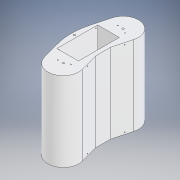
# Autodesk Inventor part: TA001
Saved by Autodesk Inventor 2017 SP1 (Build 210196100, 196)
## iProperties
Created: 2017-09-22
Part Number: TA001
Material: ABS Plastic
Document SubType Name: Modeling
Designer: Zach
Density: 1.06 g/cm^3
Appearance: CR White
Author: Zach
Autodesk Inventor part; units mm, degrees
ref_plane "YZ Plane" through (0, 0, 0) normal (1, 0, 0) x (0, 1, 0)
ref_plane "XZ Plane" through (0, 0, 0) normal (0, 1, 0) x (-1, 0, 0)
ref_plane "XY Plane" through (0, 0, 0) normal (0, 0, 1) x (1, 0, 0)
sketch "Sketch2" plane through (0, 0, 0) normal (0, 1, 0) x (-1, 0, 0)
  circle A0 centre (0, 0) radius 80 construction
  line L0 (77.2741, 20.7055) -> (103.156, -75.8871)
  line L1 (-77.2741, -20.7055) -> (-51.3922, -117.2981)
  line L2 (103.156, -75.8871) -> (-51.3922, -117.2981) construction
  line L3 (103.156, -75.8871) -> (103.156, -235.8871) construction
  line L4 (103.156, -235.8871) -> (-51.3922, -194.476) construction
  line L5 (-51.3922, -117.2981) -> (-51.3922, -194.476)
  circle A1 centre (0, -311.7741) radius 80 construction
  line L6 (-51.3922, -194.476) -> (-77.2741, -291.0686)
  line L7 (103.156, -235.8871) -> (77.2741, -332.4796)
  arc A2 (77.2741, 20.7055) -> (-77.2741, -20.7055) centre (0, 0) ccw
  arc A3 (-77.2741, -291.0686) -> (77.2741, -332.4796) centre (0, -311.7741) ccw
  circle A4 centre (0, 0) radius 5.25
  circle A5 centre (0, -311.7741) radius 5.25
  line L8 (83.156, -49.3871) -> (-29.844, -49.3871)
  line L9 (-29.844, -49.3871) -> (-29.844, -262.3871)
  line L10 (-29.844, -262.3871) -> (83.156, -262.3871)
  line L11 (83.156, -262.3871) -> (83.156, -49.3871)
  arc A6 (103.156, -235.8871) -> (103.156, -75.8871) centre (-201.516, -155.8871) ccw
  circle A7 centre (98.32, -155.8871) radius 5.25
  point P0 (103.156, -155.8871)
  point P1 (83.156, -155.8871)
  dimension "d0" = 160
  dimension "d1" = 100
  dimension "d2" = 100
  dimension "d3" = 160
  dimension "d4" = 160
  dimension "d5" = 160
  dimension "d6" = 75
  dimension "d7" = 75
  dimension "d8" = 160
  dimension "d9" = 100
  dimension "d10" = 100
  dimension "d11" = 10.5
  dimension "d12" = 10.5
  dimension "d13" = 113
  dimension "d14" = 213
  dimension "d15" = 20
  dimension "d39" = 315
  dimension "d40" = 10.5
  dimension "d41" = 15.164
  constraints: 24 end point, 10 point on circle, 8 centre point, 8 tangent, 4 coincident, 2 horizontal alignment, 2 midpoint, 2 parallel, 1 horizontal, 1 perpendicular, 1 vertical
  measures "d0" diameter of A0
  measures "d1" distance of L0.end L0.start
  measures "d2" distance of L1.end L1.start
  measures "d3" distance of L0.end L1.end
  measures "d4" distance of L0.end L3.end
  measures "d5" distance of L3.end L4.end
  measures "d6" angle of L3 L2
  measures "d7" angle of L3 L4
  measures "d8" diameter of A1
  measures "d9" distance of L4.end L6.end
  measures "d10" distance of L3.end L7.end
  measures "d11" diameter of A4
  measures "d12" diameter of A5
  measures "d13" distance of L10.end L9.end
  measures "d14" distance of L9.end L8.end
  measures "d15" distance between parallel lines of L3 L11
  measures "d39" radius of A6
  measures "d40" diameter of A7
  measures "d41" distance from line of L11 A7.centre
extrude "Extrusion1" add sketch "Sketch2" along normal blind 415 contours L0 A6 L7 A3 L6 L5 L1 A2 | A7
sketch "Sketch4" plane through (0, 0, 0) normal (1, 0, 0) x (0, 1, 0)
  line L0 (241.1371, 0) -> (230.6371, 0) construction
  line L1 (215.1815, 0) -> (315.8871, 0) construction
  line L2 (415, -306.5241) -> (415, -317.0241) projected
  line L3 (0, -317.0241) -> (0, -306.5241) projected
  line L4 (415, 5.25) -> (415, -5.25) projected
  line L5 (0, -5.25) -> (0, 5.25) projected
  line L6 (0, -306.5241) -> (415, -306.5241) construction
  line L7 (0, -317.0241) -> (415, -317.0241) construction
  line L8 (0, -5.25) -> (415, -5.25) construction
  line L9 (0, 5.25) -> (415, 5.25) construction
  line L10 (10, -322.5241) -> (40, -322.5241)
  line L11 (40, -322.5241) -> (40, -301.0241)
  line L12 (40, -301.0241) -> (10, -301.0241)
  line L13 (10, -301.0241) -> (10, -322.5241)
  line L14 (40, -10.75) -> (10, -10.75)
  line L15 (10, -10.75) -> (10, 10.75)
  line L16 (10, 10.75) -> (40, 10.75)
  line L17 (40, 10.75) -> (40, -10.75)
  line L18 (80, -322.5241) -> (110, -322.5241)
  line L19 (110, -322.5241) -> (110, -301.0241)
  line L20 (110, -301.0241) -> (80, -301.0241)
  line L21 (80, -301.0241) -> (80, -322.5241)
  line L22 (80, -10.75) -> (110, -10.75)
  line L23 (110, -10.75) -> (110, 10.75)
  line L24 (110, 10.75) -> (80, 10.75)
  line L25 (80, 10.75) -> (80, -10.75)
  point P0 (10, -311.7741)
  point P1 (0, -311.7741)
  point P2 (10, 0)
  point P3 (0, 0)
  dimension "d42" = 30
  dimension "d43" = 21.5
  dimension "d44" = 30
  dimension "d45" = 21.5
  dimension "d46" = 10
  dimension "d47" = 30
  dimension "d48" = 21.5
  dimension "d49" = 40
  dimension "d50" = 30
  dimension "d51" = 21.5
  constraints: 36 end point, 8 parallel, 4 horizontal, 4 horizontal alignment, 4 midpoint, 4 perpendicular, 1 point on line, 1 vertical alignment
  measures "d42" distance of L12.end L11.end
  measures "d43" distance of L11.end L10.end
  measures "d44" distance of L15.end L16.end
  measures "d45" distance of L14.end L15.end
  measures "d46" distance of point (0, -311.774) point (10, -311.774)
  measures "d47" distance of L20.end L19.end
  measures "d48" distance of L19.end L18.end
  measures "d49" distance between parallel lines of L11 L21
  measures "d50" distance of L24.end L23.end
  measures "d51" distance of L23.end L22.end
extrude "Extrusion3" cut sketch "Sketch4" against normal blind 113.156 and the other way blind 20
sketch "Sketch5" plane through (29.844, 0, -49.3871) normal (-1, 0, 0) x (0, 0, 1)
  line L0 (0, 0) -> (-213, 0) construction
  line L1 (0, 0) -> (0, 415) construction
  line L2 (-213, 415) -> (0, 415) construction
  line L3 (-213, 0) -> (-213, 415) construction
  line L4 (-67.911, 0) -> (28.6815, 0) construction
  line L5 (0, 415) -> (-19, 415) construction
  line L6 (-19, 415) -> (-19, 0) construction
  line L7 (-19, 0) -> (0, 0) construction
  line L8 (0, 0) -> (0, 415) construction
  line L9 (-145.089, 415) -> (-241.6815, 415) construction
  line L10 (-213, 0) -> (-194, 0) construction
  line L11 (-194, 0) -> (-194, 415) construction
  line L12 (-194, 415) -> (-213, 415) construction
  line L13 (-213, 415) -> (-213, 0) construction
  circle A0 centre (-203.5, 405) radius 2.5
  circle A1 centre (-203.5, 10) radius 2.5
  circle A2 centre (-9.5, 405) radius 2.5
  circle A3 centre (-9.5, 10) radius 2.5
  point P0 (49.3871, 0)
  point P1 (-203.5, 0)
  point P2 (-203.5, 415)
  point P3 (-9.5, 0)
  point P4 (-9.5, 415)
  dimension "d52" = 19
  dimension "d53" = 19
  dimension "d54" = 5
  dimension "d55" = 10
  dimension "d56" = 5
  dimension "d57" = 10
  dimension "d58" = 5
  dimension "d59" = 5
  dimension "d60" = 10
  dimension "d61" = 10
  constraints: 16 end point, 4 centre point, 4 midpoint, 4 parallel, 4 vertical alignment, 2 horizontal, 2 perpendicular, 2 point on line
  measures "d52" distance of L7.end L6.end
  measures "d53" distance of L12.end L11.end
  measures "d54" diameter of A0
  measures "d55" distance from line of L2 A0.centre
  measures "d56" diameter of A1
  measures "d57" distance from line of L10 A1.centre
  measures "d58" diameter of A2
  measures "d59" diameter of A3
  measures "d60" distance from line of L5 A2.centre
  measures "d61" distance from line of L0 A3.centre
extrude "Extrusion4" cut sketch "Sketch5" along normal through all both and the other way through all
sketch "Sketch6" plane through (0, 415, 0) normal (0, 1, 0) x (1, 0, 0)
  line L0 (-28.5041, 0.1269) -> (24.6218, 14.362) construction
  line L1 (-103.156, 75.8871) -> (-77.2741, -20.7055) construction
  line L2 (-77.2741, -20.7055) -> (-103.156, 75.8871) construction
  line L3 (-103.156, 75.8871) -> (51.3922, 117.2981) construction
  line L4 (-25.8819, 96.5926) -> (-1.9411, 7.2444) construction
  circle A0 centre (-28.5041, 0.1269) radius 2.5
  circle A1 centre (24.6218, 14.362) radius 2.5
  line L5 (-103.156, 235.8871) -> (-77.2741, 332.4796) construction
  line L6 (51.3922, 194.476) -> (77.2741, 291.0686) construction
  line L7 (-103.156, 235.8871) -> (51.3922, 194.476) construction
  line L8 (-25.8819, 215.1815) -> (-1.9411, 304.5297) construction
  line L9 (24.6218, 297.4122) -> (-28.5041, 311.6472) construction
  circle A2 centre (-28.5041, 311.6472) radius 2.5
  circle A3 centre (24.6218, 297.4122) radius 2.5
  point P0 (0, 0)
  dimension "d64" = 55
  dimension "d65" = 92.5
  dimension "d66" = 5
  dimension "d67" = 5
  dimension "d68" = 92.5
  dimension "d69" = 5
  dimension "d70" = 5
  dimension "d71" = 55
  constraints: 12 end point, 6 perpendicular, 5 coincident, 4 centre point, 4 midpoint
  measures "d64" distance of L0.start L0.end
  measures "d65" distance between parallel lines of L3 L0
  measures "d66" diameter of A0
  measures "d67" diameter of A1
  measures "d68" distance of L8.end L8.start
  measures "d69" diameter of A2
  measures "d70" diameter of A3
  measures "d71" distance of L9.start L9.end
extrude "Extrusion5" cut sketch "Sketch6" against normal blind 25
sketch "Sketch7" plane through (0, 415, 0) normal (0, 1, 0) x (1, 0, 0)
  circle A0 centre (-98.32, 155.8871) radius 5.25
  line L0 (-83.156, 49.3871) -> (-83.156, 262.3871) projected
  point P0 (0, 0)
  point P1 (-83.156, 155.8871)
  dimension "d76" = 10.5
  dimension "d77" = 15.164
  constraints: 1 centre point, 1 horizontal alignment, 1 midpoint
  measures "d76" diameter of A0
  measures "d77" distance from line of L0 A0.centre
extrude "Extrusion6" cut sketch "Sketch7" against normal through all
body "Solid1"
